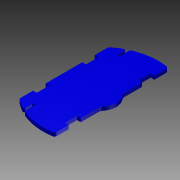
# Autodesk Inventor part: OpenROV 2.3 Dev EChassis Pivot Plate
Saved by Autodesk Inventor 2012 (Build 160160000, 160)
## iProperties
Created: 2011-12-20
Part Number: OpenROV 2.3 Dev EChassis Pivot Plate
Document SubType Name: Modeling
Designer: user
Density: 1 g/cm^3
Material: Default
Author: user
Autodesk Inventor part; units mm, degrees
ref_plane "YZ Plane" through (0, 0, 0) normal (1, 0, 0) x (0, 1, 0)
ref_plane "XZ Plane" through (0, 0, 0) normal (0, 1, 0) x (-1, 0, 0)
ref_plane "XY Plane" through (0, 0, 0) normal (0, 0, 1) x (1, 0, 0)
sketch "Sketch1" plane through (0, 0, 0) normal (0, 0, 1) x (1, 0, 0)
  line L0 (5.75, 25) -> (8.75, 25)
  line L1 (8.75, 35) -> (5.75, 35)
  line L2 (5.75, 35) -> (5.75, 25)
  line L3 (5.75, -25) -> (8.75, -25)
  line L4 (8.75, -35) -> (5.75, -35)
  line L5 (5.75, -35) -> (5.75, -25)
  arc A0 (9.8214, -7.7404) -> (9.8214, 7.7244) centre (0, -0.008) ccw
  line L6 (8.75, 25) -> (8.75, 10.8173)
  line L7 (8.75, -25) -> (8.75, -10.8333)
  arc A1 (8.75, 10.8173) -> (9.8214, 7.7244) centre (13.75, 10.8173) ccw
  arc A2 (9.8214, -7.7404) -> (8.75, -10.8333) centre (13.75, -10.8333) ccw
  line L8 (8.75, 35) -> (8.75, 44.4829)
  line L9 (8.75, -35) -> (8.75, -44.4989)
  line L10 (-30, 24.992) -> (-27, 24.992)
  line L11 (-27, 24.992) -> (-27, 14.992)
  line L12 (-27, 14.992) -> (-30, 14.992)
  line L13 (-30, -15.008) -> (-27, -15.008)
  line L14 (-27, -15.008) -> (-27, -25.1747)
  line L15 (-27, -25.1747) -> (-30, -25.1747)
  line L16 (-32, 25) -> (-32, 24.992)
  line L17 (-30, 14.992) -> (-30, -15.008)
  arc A3 (7.05, -46.4763) -> (8.75, -44.4989) centre (6.75, -44.4989) ccw
  arc A4 (8.75, 44.4829) -> (7.05, 46.4602) centre (6.75, 44.4829) ccw
  arc A5 (-21, 34.992) -> (-19, 34.992) centre (-20, 34.992) ccw
  arc A6 (-19, -35.1747) -> (-21, -35.1747) centre (-20, -35.1747) ccw
  line L18 (-21, 34.992) -> (-21, 40.39)
  line L19 (-19, 34.992) -> (-19, 42.324)
  line L20 (-21, -35.1747) -> (-21, -40.406)
  line L21 (-19, -35.1747) -> (-19, -42.34)
  arc A7 (-29.2444, -36.8015) -> (-22.4783, -41.2842) centre (0, -0.008) ccw
  arc A8 (-18.3913, -43.2603) -> (7.05, -46.4763) centre (0, -0.008) ccw
  arc A9 (7.05, 46.4602) -> (-18.3913, 43.2443) centre (0, -0.008) ccw
  arc A10 (-22.4783, 41.2682) -> (-29.2444, 36.7855) centre (0, -0.008) ccw
  arc A11 (-21, 40.39) -> (-22.4783, 41.2682) centre (-22, 40.39) ccw
  arc A12 (-18.3913, 43.2443) -> (-19, 42.324) centre (-18, 42.324) ccw
  arc A13 (-22.4783, -41.2842) -> (-21, -40.406) centre (-22, -40.406) ccw
  arc A14 (-19, -42.34) -> (-18.3913, -43.2603) centre (-18, -42.34) ccw
  line L22 (-30, 24.992) -> (-30, 35.2198)
  line L23 (-30, -25.1747) -> (-30, -35.2358)
  arc A15 (-29.2444, 36.7855) -> (-30, 35.2198) centre (-28, 35.2198) ccw
  arc A16 (-30, -35.2358) -> (-29.2444, -36.8015) centre (-28, -35.2358) ccw
  point P0 (8.75, 8.9188)
  point P1 (8.75, -8.9348)
  point P2 (8.75, 46.1703)
  point P3 (8.75, -46.1863)
  point P4 (-21, 42.0396)
  point P5 (-19, 42.9804)
  point P6 (-21, -42.0556)
  point P7 (-19, -42.9964)
  point P8 (-30, 36.1721)
  point P9 (-30, -36.1881)
  dimension "d13" = 10
  dimension "d17" = 10
  dimension "d70" = 3
  dimension "d72" = 3
  dimension "d107" = 25
  dimension "d108" = 5
  dimension "d114" = 10
  dimension "d115" = 10.1667
  dimension "d116" = 15
  dimension "d117" = 15
  dimension "d119" = 2
  dimension "d120" = 2
  dimension "d122" = 10
  dimension "d124" = 10
  dimension "d125" = 1
  dimension "d126" = 30
  dimension "d127" = 27
  dimension "d128" = 27
  dimension "d130" = 30
  dimension "d131" = 30
  dimension "d132" = 2
  constraints: 48 end point, 42 point on circle, 22 tangent, 17 centre point, 12 parallel, 11 point on line, 5 equal radius, 4 horizontal, 3 collinear, 2 perpendicular, 1 coincident
  measures "d13" distance of L1.end L0.start
  measures "d17" distance of L4.end L3.start
  measures "d70" distance of L1.start L1.end
  measures "d72" distance of L4.start L4.end
  measures "d107" diameter of A0
  measures "d108" radius of A1
  measures "d114" distance of L10.end L11.end
  measures "d115" distance of L13.end L14.end
  measures "d116" distance from line of A0.centre L13
  measures "d117" distance from line of L12 A0.centre
  measures "d119" diameter of A5
  measures "d120" diameter of A6
  measures "d122" distance from line of L10 A5.centre
  measures "d124" distance from line of L15 A6.centre
  measures "d125" radius of A11
  measures "d126" distance from line of A0.centre L17
  measures "d127" distance from line of A0.centre L14
  measures "d128" distance from line of A0.centre L11
  measures "d130" distance from line of A0.centre L23
  measures "d131" distance from line of A0.centre L22
  measures "d132" radius of A15
extrude "Extrusion6" add sketch "Sketch1" along normal blind 3
body "Solid6"
